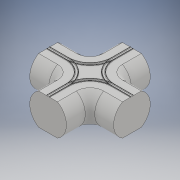
# Autodesk Inventor part: S corridor
Saved by Autodesk Inventor 2017 (Build 210142000, 142)
## iProperties
Created: 2018-03-04
Part Number: S corridor
Material: Generic
Document SubType Name: Modeling
Designer: Braxton
Density: 1 g/cm^3
Appearance: Default
Author: Braxton
Autodesk Inventor part; units mm, degrees
ref_plane "YZ Plane" through (0, 0, 0) normal (1, 0, 0) x (0, 1, 0)
ref_plane "XZ Plane" through (0, 0, 0) normal (0, 1, 0) x (-1, 0, 0)
sketch "Sketch1" plane through (0, 0, 0) normal (1, 0, 0) x (0, 1, 0)
  line L0 (91.0167, 0) -> (87.8622, 0) construction
  line L1 (87.8622, 7.4083) -> (86.2542, 7.4083)
  line L2 (87.8622, -7.4083) -> (86.2542, -7.4083)
  line L3 (84.6667, 8.9958) -> (84.6667, -8.9958) construction
  arc A0 (84.6667, -4.0844) -> (86.9132, -6.35) centre (86.9324, -4.0844) ccw
  line L4 (84.6873, -6.3294) -> (87.8622, -3.1545) construction
  line L5 (87.8622, -6.35) -> (87.8622, 0) construction
  line L6 (87.8622, -6.35) -> (86.9132, -6.35)
  arc A1 (87.8622, -6.35) -> (84.6667, -3.1545) centre (84.6873, -6.3294) ccw construction
  line L7 (87.8622, -7.4083) -> (87.8622, -6.35)
  arc A2 (86.2542, -7.4083) -> (84.6667, -8.9958) centre (86.2542, -8.9958) ccw
  line L8 (84.6667, -4.0844) -> (84.6667, 0)
  arc A3 (84.6667, 8.9958) -> (86.2542, 7.4083) centre (86.2542, 8.9958) ccw
  line L9 (87.8622, 6.35) -> (87.8622, 7.4083)
  line L10 (84.6667, 8.9958) -> (84.6667, 50.8)
  line L11 (-84.6667, 50.8) -> (-84.6667, -50.8)
  arc A4 (84.6667, 50.8) -> (-84.6667, 50.8) centre (0, 0) ccw construction
  arc A5 (-84.6667, -50.8) -> (84.6667, -50.8) centre (0, 0) ccw
  line L12 (84.6667, -8.9958) -> (84.6667, -50.8)
  line L13 (84.6667, 0) -> (87.8622, 0) construction
  line L14 (84.6667, 4.0844) -> (84.6667, 0)
  line L15 (87.8622, 6.35) -> (87.8622, 0) construction
  line L16 (84.6873, 6.3294) -> (87.8622, 3.1545) construction
  arc A6 (84.6667, 3.1545) -> (87.8622, 6.35) centre (84.6873, 6.3294) ccw construction
  line L17 (87.8622, 6.35) -> (86.9132, 6.35)
  arc A7 (86.9132, 6.35) -> (84.6667, 4.0844) centre (86.9324, 4.0844) ccw
  line L18 (84.6667, 0) -> (-84.6667, 0)
  dimension "d196" = 101.6
  dimension "d197" = 14.8167
  dimension "d198" = 98.7374
  dimension "d199" = 98.7374
  dimension "d200" = 43.3917
  dimension "d201" = 1.5875
  dimension "d202" = 1.5875
  dimension "d203" = 41.8042
  dimension "d204" = 6.35
  dimension "d205" = 3.175
  dimension "d206" = 2.2657
  dimension "d207" = 2.2466
  dimension "d208" = 45
  dimension "d209" = 84.6667
  constraints: 38 end point, 19 point on circle, 10 symmetric about line, 8 centre point, 7 point on line, 5 collinear, 4 perpendicular, 3 coincident, 2 tangent, 1 midpoint, 1 parallel, 1 vertical, 4 other
  measures "d196" distance of L10.end L12.end
  measures "d197" distance of L1.start L2.start
  measures "d198" radius of A4
  measures "d199" radius of A5
  measures "d200" distance from line of L10.end L1
  measures "d201" distance from line of L12.start L2
  measures "d202" radius of A2
  measures "d203" distance of L12.start L12.end
  measures "d204" distance of L13.end L15.start
  measures "d205" distance of L15.start L16.start
  measures "d206" radius of A7
  measures "d207" horizontal distance of L14.start L17.end
  measures "d208" angle of L15 L16
  measures "d209" distance from line of L11 point (0, 0)
extrude "corridor eighth" add sketch "Sketch1" against normal blind 101.6
ref_plane "Work Plane1" through (0, 0, -124.1375) normal (0, 0, 1) x (1, 0, 0)
sketch "Sketch7" plane through (0, 0, 0) normal (0, 1, 0) x (-1, 0, 0)
  line L0 (-25.4, -124.1375) -> (-25.4, -225.7375) construction
  line L1 (0, -98.7375) -> (0, -50.8) projected
  arc A0 (0, -98.7375) -> (-25.4, -124.1375) centre (0, -124.1375) ccw
  line L2 (0, -98.7375) -> (101.6, -98.7375) projected
  dimension "d160" = 101.6
  dimension "d211" = 25.4
  constraints: 2 end point, 2 point on circle, 2 tangent, 1 centre point, 1 vertical
  measures "d160" distance of L0.start L0.end
  measures "d211" radius of A0
sketch "Sketch22" plane through (0, 0, 0) normal (1, 0, 0) x (0, 0, -1)
  arc A0 (4.0844, 84.6667) -> (6.35, 86.9132) centre (4.0844, 86.9324) ccw projected
  line L0 (6.35, 87.8622) -> (7.4083, 87.8622) projected
  line L1 (6.35, 86.9132) -> (6.35, 87.8622)
  line L2 (6.35, 87.8622) -> (7.4083, 87.8622)
  line L3 (7.4083, 87.8622) -> (7.4083, 86.2542) projected
  line L4 (7.4083, 87.8622) -> (7.4083, 86.2542)
  line L5 (8.9958, 84.6667) -> (50.8, 84.6667) projected
  line L6 (8.9958, 84.6667) -> (50.8, 84.6667)
  line L7 (0, 84.6667) -> (4.0844, 84.6667) projected
  line L8 (4.0844, 84.6667) -> (0, 84.6667)
  arc A1 (4.0844, 84.6667) -> (6.35, 86.9132) centre (4.0844, 86.9324) ccw
  arc A2 (7.4083, 86.2542) -> (8.9958, 84.6667) centre (8.9958, 86.2542) ccw
  arc A3 (50.8, -84.6667) -> (50.8, 84.6667) centre (0, 0) ccw projected
  arc A4 (50.8, 84.6667) -> (50.8, 84.6667) centre (0, 0) ccw
  line L9 (50.8, -84.6667) -> (0, -84.6667) projected
  arc A5 (50.8, -84.6667) -> (50.8, 84.6667) centre (0, 0) ccw
  line L10 (50.8, -84.6667) -> (0, -84.6667)
  line L11 (0, -84.6667) -> (0, 84.6667) construction
  arc A6 (7.4083, 86.2542) -> (8.9958, 84.6667) centre (8.9958, 86.2542) ccw projected
  arc A7 (-6.35, 86.9132) -> (-4.0844, 84.6667) centre (-4.0844, 86.9324) ccw
  line L12 (-6.35, 87.8622) -> (-7.4083, 87.8622)
  line L13 (-6.35, 86.9132) -> (-6.35, 87.8622)
  line L14 (-7.4083, 87.8622) -> (-7.4083, 86.2542)
  line L15 (0, 84.6667) -> (-4.0844, 84.6667)
  arc A8 (-8.9958, 84.6667) -> (-7.4083, 86.2542) centre (-8.9958, 86.2542) ccw
  line L16 (-8.9958, 84.6667) -> (-8.9958, -84.6667)
  line L17 (-8.9958, -84.6667) -> (0, -84.6667)
  constraints: 24 end point, 10 point on circle, 8 symmetric about line, 5 centre point, 4 concentric, 3 perpendicular, 2 collinear, 2 parallel, 1 horizontal, 6 other
sweep "Sweep4" add profiles "Sketch22" path "Sketch7" path curves A0 contours A0 L1 L0 L3 A2 L5 A3 L9 L17 L16 A8 L14 L12 L13 A7 L15 L7
ref_plane "mirror plane YZ" through (124.1375, 104.4021, -124.1375) normal (1, 0, 0) x (0, 1, 0)
sketch "Sketch23" plane through (133.1333, -84.6667, -124.1375) normal (0, 0, -1) x (-1, 0, 0)
  arc A0 (13.0802, 169.3333) -> (15.3458, 171.5799) centre (13.0802, 171.599) ccw projected
  line L0 (133.1333, 169.3333) -> (4.9115, 169.3333) construction
  line L1 (13.0802, 169.3333) -> (4.9115, 169.3333)
  line L2 (8.9958, 169.3333) -> (8.9958, 0)
  line L3 (0, 0) -> (59.7958, 0) projected
  line L4 (8.9958, 0) -> (59.7958, 0)
  line L5 (133.1333, 171.5799) -> (15.3458, 171.5799) projected
  line L6 (15.3458, 172.5289) -> (15.3458, 171.5799) projected
  line L7 (15.3458, 171.5799) -> (15.3458, 172.5289)
  line L8 (16.4042, 170.9208) -> (16.4042, 172.5289) projected
  line L9 (15.3458, 172.5289) -> (16.4042, 172.5289)
  line L10 (16.4042, 172.5289) -> (16.4042, 170.9208)
  arc A1 (16.4042, 170.9208) -> (17.9917, 169.3333) centre (17.9917, 170.9208) ccw projected
  arc A2 (59.7958, 0) -> (59.7958, 169.3333) centre (8.9958, 84.6667) ccw projected
  line L11 (59.7958, 169.3333) -> (17.9917, 169.3333)
  arc A3 (13.0802, 169.3333) -> (15.3458, 171.5799) centre (13.0802, 171.599) ccw
  arc A4 (16.4042, 170.9208) -> (17.9917, 169.3333) centre (17.9917, 170.9208) ccw
  arc A5 (59.7958, 0) -> (59.7958, 169.3333) centre (8.9958, 84.6667) ccw
  point P0 (133.1333, 84.6667)
  constraints: 14 end point, 6 point on circle, 5 collinear, 3 centre point, 3 concentric, 1 coincident, 1 midpoint, 1 perpendicular, 1 point on line, 1 tangent, 1 vertical
extrude "corridor eighth complete" add sketch "Sketch23" along normal blind 101.6
mirror "Mirror half" about plane through (124.1375, 104.4021, -124.1375) normal (1, 0, 0) of "corridor eighth", "Sweep4", "corridor eighth complete"
mirror "Mirrorfull" about plane through (248.2749, -84.6667, 0) normal (0, 0, 1) of "corridor eighth", "Sweep4", "corridor eighth complete", "Mirror half"
sketch "Sketch24" plane through (-101.6, 84.6667, 50.8) normal (0, 1, 0) x (1, 0, 0)
  arc A0 (149.7078, 50.8) -> (225.7375, 126.8296) centre (101.6, 174.9375) ccw projected
  arc A1 (149.7078, 50.8) -> (225.7375, 126.8296) centre (101.6, 174.9375) ccw
  arc A2 (225.7375, 126.8296) -> (301.7671, 50.8) centre (349.8749, 174.9375) ccw projected
  arc A3 (225.7375, 126.8296) -> (225.7375, 126.8296) centre (305.3126, 130.3751) ccw
  arc A4 (225.7375, 126.8296) -> (301.7671, 50.8) centre (349.8749, 174.9375) ccw
  arc A5 (225.7375, -25.2296) -> (149.7078, 50.8) centre (101.6, -73.3375) ccw projected
  arc A6 (301.7671, 50.8) -> (225.7375, -25.2296) centre (349.8749, -73.3375) ccw projected
  arc A7 (225.7375, -25.2296) -> (149.7078, 50.8) centre (101.6, -73.3375) ccw
  arc A8 (301.7671, 50.8) -> (225.7375, -25.2296) centre (349.8749, -73.3375) ccw
  point P0 (101.6, 50.8)
  constraints: 8 point on circle, 4 centre point, 4 concentric, 5 other
extrude "hole fill in" add sketch "Sketch24" against normal up to surface (169.3333 mm away) contours A0 A3 A6 A5 | A2 A3 picked at (253.5972, 78.6597)
equation "\"d5\" = -0.5 * d2"
equation "\"d2\" = 248.274904"
body "Solid1"
